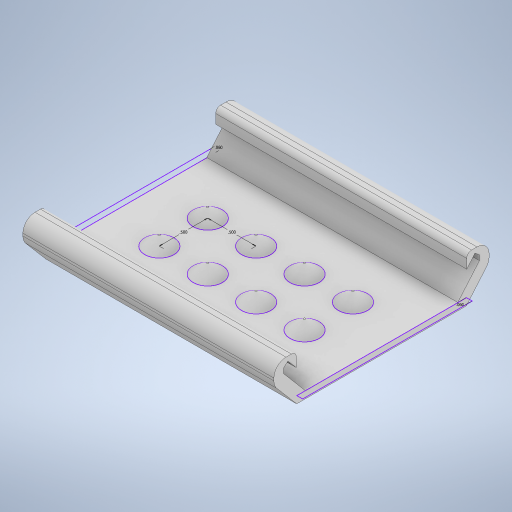
# Autodesk Inventor part: ControllerClamp
Saved by Autodesk Inventor 2024 (Build 280153000, 153)
## iProperties
Created: 2024-03-27
Part Number: ControllerClamp
Material: Generic
Document SubType Name: Modeling
Designer: bbbmi
Density: 1 g/cm^3
Appearance: Default
Author: bbbmi
Autodesk Inventor part; units mm, degrees
ref_plane "YZ Plane" through (0, 0, 0) normal (1, 0, 0) x (0, 1, 0)
ref_plane "XZ Plane" through (0, 0, 0) normal (0, 1, 0) x (-1, 0, 0)
ref_plane "XY Plane" through (0, 0, 0) normal (0, 0, 1) x (1, 0, 0)
sketch "Sketch1" plane through (0, 0, 0) normal (0, 1, 0) x (-1, 0, 0)
  line L0 (24.9723, 27.098) -> (-43.9316, 27.098)
  line L1 (-43.9316, 27.098) -> (-43.9316, -17.4091)
  line L2 (-43.9316, -17.4091) -> (24.9723, -17.4091)
  line L3 (24.9723, -17.4091) -> (24.9723, 27.098)
  circle A0 centre (9.5704, -1.5056) radius 3.81
  circle A1 centre (-3.1296, -1.5056) radius 3.81
  circle A2 centre (-15.8296, -1.5056) radius 3.81
  circle A3 centre (-28.5296, -1.5056) radius 3.81
  circle A4 centre (9.5704, 11.1944) radius 3.81
  circle A5 centre (-3.1296, 11.1944) radius 3.81
  circle A6 centre (-15.8296, 11.1944) radius 3.81
  circle A7 centre (-28.5296, 11.1944) radius 3.81
  line L4 (24.9723, -17.4091) -> (23.4483, -17.4091)
  line L5 (23.4483, -17.4091) -> (23.4483, 27.098)
  line L6 (-43.9316, -17.4091) -> (-42.4076, -17.4091)
  line L7 (-42.4076, -17.4091) -> (-42.4076, 27.098)
  point P0 (0, 0)
  dimension "d3" = 12.7
  dimension "d6" = 12.7
  dimension "d9" = 1.524
  dimension "d10" = 1.524
  constraints: 16 end point, 8 centre point, 4 point on line, 2 perpendicular, 1 horizontal, 1 vertical, 14 other
  measures "d3" distance of A0.centre A1.centre
  measures "d6" distance of A0.centre A4.centre
  measures "d9" distance of L2.end L4.end
  measures "d10" distance of L2.start L6.end
extrude "Extrusion1" add sketch "Sketch1" against normal blind 1.905 contours L5 L2 L7 L0 | A0 | A1 | A2 | A3 | A4 | A5 | A6 | A7
extrude "Extrusion2" add sketch "Sketch1" along normal blind 2.54 contours A0 | A1 | A2 | A3 | A4 | A5 | A6 | A7
chamfer "Chamfer1" distance 3.556 distance2 2.54 1 edges at (-5.7604, 2.54, 11.1944) measured on face at (-7.8424, 2.54, 10.6775)
chamfer "Chamfer2" distance 3.556 distance2 2.54 1 edges at (-5.7604, 2.54, -1.5056) measured on face at (-9.9176, 2.54, -0.5901)
chamfer "Chamfer3" distance 3.556 distance2 2.54 1 edges at (6.9396, 2.54, -1.5056) measured on face at (2.4763, 2.54, -0.5901)
chamfer "Chamfer4" distance 3.556 distance2 2.54 1 edges at (19.6396, 2.54, -1.5056) measured on face at (16.7802, 2.54, -2.3477)
chamfer "Chamfer5" distance 3.556 distance2 2.54 1 edges at (32.3396, 2.54, -1.5056) measured on face at (28.1824, 2.54, -0.5901)
chamfer "Chamfer6" distance 3.556 distance2 2.54 1 edges at (6.9396, 2.54, 11.1944) measured on face at (2.382, 2.54, 9.9337)
chamfer "Chamfer7" distance 3.556 distance2 2.54 1 edges at (19.6396, 2.54, 11.1944) measured on face at (16.7802, 2.54, 10.3523)
chamfer "Chamfer8" distance 3.556 distance2 2.54 1 edges at (32.3396, 2.54, 11.1944) measured on face at (28.1824, 2.54, 12.1099)
sketch "Sketch2" plane through (42.4076, 0, 27.098) normal (1, 0, 0) x (0, 0, -1)
  line L0 (19.1798, 6.2965) -> (19.1798, 7.6808)
  arc A0 (21.1991, 9.7001) -> (19.1798, 7.6808) centre (21.1991, 7.6808) ccw
  line L1 (21.1991, 9.7001) -> (26.1711, 9.7001)
  arc A1 (27.8729, 7.9983) -> (26.1711, 9.7001) centre (26.1711, 7.9983) ccw
  line L2 (27.8729, 7.9983) -> (27.8729, 6.2965)
  arc A2 (27.2379, 5.6615) -> (27.8729, 6.2965) centre (27.2379, 6.2965) ccw
  line L3 (27.2379, 5.6615) -> (19.8148, 5.6615)
  arc A3 (19.1798, 6.2965) -> (19.8148, 5.6615) centre (19.8148, 6.2965) ccw
  line L4 (26.8541, 21.209) -> (26.8541, 19.8247)
  arc A4 (24.8348, 17.8054) -> (26.8541, 19.8247) centre (24.8348, 19.8247) ccw
  line L5 (24.8348, 17.8054) -> (19.8628, 17.8054)
  arc A5 (18.161, 19.5072) -> (19.8628, 17.8054) centre (19.8628, 19.5072) ccw
  line L6 (18.161, 19.5072) -> (18.161, 21.209)
  arc A6 (18.796, 21.844) -> (18.161, 21.209) centre (18.796, 21.209) ccw
  line L7 (18.796, 21.844) -> (26.2191, 21.844)
  arc A7 (26.8541, 21.209) -> (26.2191, 21.844) centre (26.2191, 21.209) ccw
  line L8 (44.5071, 3.302) -> (0, 3.302)
  line L9 (44.5071, 3.302) -> (47.4281, 6.7381)
  line L10 (47.4281, 6.7381) -> (47.4281, 7.7839)
  line L11 (44.5071, 7.7839) -> (44.5071, 27.94)
  line L12 (42.6021, 27.94) -> (44.5071, 27.94)
  line L13 (42.6021, 26.9875) -> (42.6021, 27.94)
  line L14 (42.6021, 26.9875) -> (43.5546, 26.9875)
  line L15 (43.5546, 26.035) -> (43.5546, 26.9875)
  line L16 (0.9525, 26.035) -> (43.5546, 26.035)
  line L17 (0.9525, 26.035) -> (0.9525, 26.9875)
  line L18 (0.9525, 26.9875) -> (1.905, 26.9875)
  line L19 (1.905, 26.9875) -> (1.905, 27.94)
  line L20 (0, 27.94) -> (1.905, 27.94)
  line L21 (0, 7.7839) -> (0, 27.94)
  line L22 (0, 7.7839) -> (-2.921, 7.7839)
  line L23 (-2.921, 7.7839) -> (-2.921, 6.7381)
  line L24 (-2.921, 6.7381) -> (0, 3.302)
  line L25 (0, 0) -> (44.5071, 0) projected
  line L26 (0, -1.905) -> (-5.2131, 4.2274)
  line L27 (0, 3.302) -> (2.807, 0)
  line L28 (2.807, 0) -> (2.241, 0)
  line L29 (2.241, 0) -> (-3.429, 6.6699)
  line L30 (-2.921, 6.7381) -> (-3.429, 6.7381)
  line L31 (-3.429, 6.7381) -> (-3.429, 6.6699)
  line L32 (-3.429, 6.7381) -> (-3.429, 7.7839)
  line L33 (-3.429, 7.7839) -> (-3.429, 8.2919)
  line L34 (-2.921, 7.7839) -> (-1.651, 7.7839)
  line L35 (-1.651, 7.7839) -> (0, 5.8417)
  line L36 (-5.969, 8.2919) -> (-5.969, 5.6615)
  line L37 (-5.8869, 5.0201) -> (-5.969, 5.1167)
  line L38 (-5.969, 5.6615) -> (-5.969, 6.2838)
  line L39 (0, 6.2616) -> (-2.286, 8.9508)
  line L40 (-2.286, 8.9508) -> (-3.429, 7.9791)
  line L41 (-0.1085, 6.3892) -> (-0.1085, 8.8286)
  line L42 (-1.3785, 10.0986) -> (-2.794, 10.0986)
  line L43 (-5.969, 6.9236) -> (-5.969, 8.2919)
  arc A8 (-2.794, 10.0986) -> (-5.969, 6.9236) centre (-2.794, 6.9236) ccw
  line L44 (47.4281, 7.7839) -> (47.4281, 6.7381)
  line L45 (47.4281, 6.7381) -> (47.9361, 6.7381)
  line L46 (47.9361, 6.7381) -> (47.9361, 6.6699)
  line L47 (47.9361, 6.7381) -> (47.9361, 7.7839)
  line L48 (47.9361, 7.7839) -> (47.9361, 8.2919)
  line L49 (46.7931, 8.9508) -> (47.9361, 7.9791)
  arc A9 (50.4761, 6.9236) -> (47.3011, 10.0986) centre (47.3011, 6.9236) ccw
  line L50 (50.4761, 6.9236) -> (50.4761, 8.2919)
  line L51 (50.4761, 8.2919) -> (50.4761, 6.2838)
  line L52 (50.4761, 5.6615) -> (50.4761, 5.1167)
  line L53 (50.394, 5.0201) -> (50.4761, 5.1167)
  line L54 (47.4281, 6.7381) -> (44.5071, 3.302)
  line L55 (41.7002, 0) -> (42.2662, 0)
  line L56 (44.6156, 6.3892) -> (44.6156, 8.8286)
  line L57 (44.5071, 3.302) -> (41.7002, 0)
  line L58 (44.5071, 6.2616) -> (46.7931, 8.9508)
  line L59 (45.8856, 10.0986) -> (47.3011, 10.0986)
  line L60 (42.2662, 0) -> (47.9361, 6.6699)
  line L61 (44.5071, -1.905) -> (49.7202, 4.2274)
  line L62 (44.5071, 0) -> (44.5071, -1.905) projected
  line L63 (0, 0) -> (0, -1.905) projected
  line L64 (0, -1.905) -> (0, 0)
  line L65 (0, 0) -> (2.241, 0)
  line L66 (44.5071, -1.905) -> (44.5071, 0)
  line L67 (44.5071, 0) -> (42.2662, 0)
  arc A10 (-5.969, 6.2838) -> (-5.2131, 4.2274) centre (-2.794, 6.2838) ccw
  arc A11 (49.7202, 4.2274) -> (50.4761, 6.2838) centre (47.3011, 6.2838) ccw
  arc A12 (-0.1085, 8.8286) -> (-1.3785, 10.0986) centre (-1.3785, 8.8286) ccw
  arc A13 (45.8856, 10.0986) -> (44.6156, 8.8286) centre (45.8856, 8.8286) ccw
  point P0 (27.098, 0)
  point P1 (2.3019, 5.207)
  point P2 (-0.1085, 10.0986)
  point P3 (58.983, -0.9263)
  point P4 (58.983, -2.8313)
  point P5 (42.2053, 5.207)
  point P6 (44.6156, 10.0986)
  point P7 (50.4761, 6.9236)
  point P8 (-1.2941, 7.7839)
  point P9 (-0.1085, 7.7839)
  dimension "d41" = 3.302
  dimension "d42" = 0.508
  dimension "d43" = 0.508
  dimension "d44" = 1.27
  dimension "d45" = 2.54
  dimension "d46" = 3.175
  dimension "d53" = 3.175
  dimension "d56" = 1.27
  constraints: 130 end point, 28 point on circle, 17 point on line, 14 centre point, 10 tangent, 6 perpendicular, 4 parallel, 4 vertical, 2 collinear, 2 equal radius, 1 horizontal
  measures "d41" distance of L25.start L27.start
  measures "d42" distance of L24.start L30.end
  measures "d43" distance of L32.end L33.end
  measures "d44" distance of L22.end L34.end
  measures "d45" distance of L33.end L36.start
  measures "d46" radius of A8
  measures "d53" radius of A10
  measures "d56" radius of A12
extrude "Extrusion3" add sketch "Sketch2" against normal up to surface (65.8559 mm away) contours L47 L48 L49 L58 L56 A13 L59 A9 L51 A11 L61 L62 L25 L60 L46 | L31 L29 L25 L63 L26 A10 L36 A8 L42 A12 L41 L22 L39 L40 L33 L32 | L22 L41 L39
body "Solid1"
